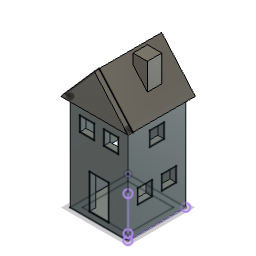
MMEZP_Domecek_2_patra v1 (Autodesk Fusion 360 design; units mm, degrees)
Autodesk Fusion 360 part; units mm, degrees
sketch "Sketch1" plane through (0, 0, 0) normal (0, 1, 0) x (1, 0, 0)
  line L0 (0, 0) -> (30, 0)
  line L1 (30, 0) -> (30, -30)
  line L2 (30, -30) -> (0, -30)
  line L3 (0, -30) -> (0, 0)
  line L4 (3.2, -3.2) -> (26.8, -3.2)
  line L5 (26.8, -3.2) -> (26.8, -26.8)
  line L6 (26.8, -26.8) -> (3.2, -26.8)
  line L7 (3.2, -26.8) -> (3.2, -3.2)
  dimension "d1" = 30
  dimension "d2" = 30
  dimension "d3" = 3.2
  dimension "d4" = 3.2
  dimension "d5" = 3.2
  dimension "d6" = 3.2
  constraint horizontal L0
  constraint vertical L1
  constraint horizontal L2
  constraint vertical L3
  constraint coincident L0.start L3.end
  constraint horizontal L4
  constraint vertical L5
  constraint horizontal L6
  constraint vertical L7
  measures "d1" distance of L0.start L0.end
  measures "d2" distance of L0.start L2.end
  measures "d3" distance of L1 L5
  measures "d4" distance of L0 L4
  measures "d5" distance of L3 L7
  measures "d6" distance of L2 L6
extrude "Extrude1" add sketch "Sketch1" along normal blind 50 makes body 1
sketch "Sketch2" plane through (0, 0, 30) normal (0, 0, 1) x (1, 0, 0)
  line L0 (0, 0) -> (30, 0)
  line L1 (30, 0) -> (30, 50)
  line L2 (30, 50) -> (0, 50)
  line L3 (0, 50) -> (0, 0)
  line L4 (10, 3.2) -> (20, 3.2)
  line L5 (20, 3.2) -> (20, 21.2)
  line L6 (20, 21.2) -> (10, 21.2)
  line L7 (10, 21.2) -> (10, 3.2)
  line L8 (5, 44) -> (12.5, 44)
  line L9 (12.5, 44) -> (12.5, 36.5)
  line L10 (12.5, 36.5) -> (5, 36.5)
  line L11 (5, 36.5) -> (5, 44)
  line L12 (17.5, 44) -> (25, 44)
  line L13 (25, 44) -> (25, 36.5)
  line L14 (25, 36.5) -> (17.5, 36.5)
  line L15 (17.5, 36.5) -> (17.5, 44)
  line L16 (0, 50) -> (-2.5, 50)
  line L17 (30, 50) -> (32.5, 50)
  line L18 (-2.5, 50) -> (15, 70)
  line L19 (15, 70) -> (32.5, 50)
  dimension "d9" = 18
  dimension "d10" = 10
  dimension "d11" = 10
  dimension "d12" = 3.2
  dimension "d13" = 7.5
  dimension "d14" = 7.5
  dimension "d15" = 5
  dimension "d16" = 6
  dimension "d17" = 7.5
  dimension "d18" = 7.5
  dimension "d19" = 5
  dimension "d20" = 6
  dimension "d51" = 2.5
  dimension "d52" = 2.5
  dimension "d53" = 17.5
  dimension "d54" = 20
  constraint horizontal L4
  constraint vertical L5
  constraint horizontal L6
  constraint vertical L7
  constraint horizontal L8
  constraint vertical L9
  constraint horizontal L10
  constraint vertical L11
  constraint horizontal L12
  constraint vertical L13
  constraint horizontal L14
  constraint vertical L15
  constraint coincident L2.end L3.start
  constraint perpendicular L3 L16
  constraint coincident L1.end L2.start
  constraint perpendicular L1 L17
  measures "d9" distance of L4.start L6.end
  measures "d10" distance of L4.start L4.end
  measures "d11" distance of L3 L7
  measures "d12" distance of L0 L4
  measures "d13" distance of L8.start L8.end
  measures "d14" distance of L8.start L10.end
  measures "d15" distance of L3 L11
  measures "d16" distance of L2 L8
  measures "d17" distance of L12.start L12.end
  measures "d18" distance of L12.start L14.end
  measures "d19" distance of L1 L13
  measures "d20" distance of L2 L12
  measures "d51" distance of L2.end L16.end
  measures "d52" distance of L1.end L17.end
  measures "d53" horizontal distance of L17.end L18.end
  measures "d54" distance of L2 L18.end
extrude "Extrude2" cut sketch "Sketch2" against normal blind 3.2 contours L4 L5 L6 L7 bodies 1
extrude "Extrude3" add sketch "Sketch1" along normal blind 3.2 contours L4 L5 L6 L7 bodies 1
extrude "Extrude4" cut sketch "Sketch2" against normal blind 3.2 contours L8 L9 L10 L11 | L12 L13 L14 L15 bodies 1
sketch "Sketch3" plane through (30, 0, 0) normal (1, 0, 0) x (0, 0, -1)
  line L0 (-30, 0) -> (0, 0)
  line L1 (0, 0) -> (0, 50)
  line L2 (0, 50) -> (-30, 50)
  line L3 (-30, 50) -> (-30, 0)
  line L4 (-25, 21.2) -> (-17.5, 21.2)
  line L5 (-17.5, 21.2) -> (-17.5, 13.7)
  line L6 (-17.5, 13.7) -> (-25, 13.7)
  line L7 (-25, 13.7) -> (-25, 21.2)
  line L8 (-12.5, 21.2) -> (-5, 21.2)
  line L9 (-5, 21.2) -> (-5, 13.7)
  line L10 (-5, 13.7) -> (-12.5, 13.7)
  line L11 (-12.5, 13.7) -> (-12.5, 21.2)
  line L12 (-30, 3.2) -> (-30, 21.2)
  line L13 (0, 0) -> (-30, 0)
  line L14 (-18.75, 44) -> (-11.25, 44)
  line L15 (-11.25, 44) -> (-11.25, 36.5)
  line L16 (-11.25, 36.5) -> (-18.75, 36.5)
  line L17 (-18.75, 36.5) -> (-18.75, 44)
  dimension "d27" = 7.5
  dimension "d28" = 7.5
  dimension "d29" = 5
  dimension "d30" = 5
  dimension "d31" = 7.5
  dimension "d32" = 7.5
  dimension "d33" = 13.7
  dimension "d34" = 13.7
  dimension "d35" = 6
  dimension "d36" = 7.5
  dimension "d37" = 7.5
  dimension "d38" = 11.25
  constraint horizontal L4
  constraint vertical L5
  constraint horizontal L6
  constraint vertical L7
  constraint horizontal L8
  constraint vertical L9
  constraint horizontal L10
  constraint vertical L11
  constraint horizontal L14
  constraint vertical L15
  constraint horizontal L16
  constraint vertical L17
  measures "d27" distance of L4.start L4.end
  measures "d28" distance of L4.start L6.end
  measures "d29" distance of L7 L12
  measures "d30" distance of L1 L9
  measures "d31" distance of L8.start L8.end
  measures "d32" distance of L8.start L10.end
  measures "d33" distance of L6 L13
  measures "d34" distance of L10 L13
  measures "d35" distance of L2 L14
  measures "d36" distance of L14.start L16.end
  measures "d37" distance of L15.end L16.end
  measures "d38" distance of L1 L15
extrude "Extrude5" cut sketch "Sketch3" against normal blind 30 contours L14 L15 L16 L17 bodies 1
extrude "Extrude6" cut sketch "Sketch3" against normal blind 30 contours L4 L5 L6 L7 | L8 L9 L10 L11 bodies 1
sketch "Sketch4" plane through (0, 50, 0) normal (0, 1, 0) x (-1, 0, 0)
  line L0 (-26.8, 26.8) -> (-3.2, 26.8)
  line L1 (-3.2, 26.8) -> (-3.2, 3.2)
  line L2 (-3.2, 3.2) -> (-26.8, 3.2)
  line L3 (-26.8, 3.2) -> (-26.8, 26.8)
  line L4 (0, 30) -> (-30, 30)
  line L5 (-30, 30) -> (-30, 0)
  line L6 (-30, 0) -> (0, 0)
  line L7 (0, 0) -> (0, 30)
  line L8 (2.5, -2.5) -> (-32.5, -2.5)
  line L9 (-32.5, -2.5) -> (-32.5, 32.5)
  line L10 (-32.5, 32.5) -> (2.5, 32.5)
  line L11 (2.5, 32.5) -> (2.5, -2.5)
  line L12 (0, 30) -> (0, 0)
  line L13 (0, 0) -> (-30, 0)
  line L14 (-30, 0) -> (-30, 30)
  line L15 (-30, 30) -> (0, 30)
  line L16 (-18.3, 8.2) -> (-25.8, 8.2)
  line L17 (-25.8, 8.2) -> (-25.8, 15.7)
  line L18 (-25.8, 15.7) -> (-18.3, 15.7)
  line L19 (-18.3, 15.7) -> (-18.3, 8.2)
  line L20 (-26.8, 26.8) -> (-3.2, 26.8)
  line L21 (-26.8, 3.2) -> (-26.8, 26.8)
  line L22 (-3.2, 3.2) -> (-26.8, 3.2)
  dimension "d43" = 2.5
  dimension "d44" = 2.5
  dimension "d45" = 2.5
  dimension "d46" = 2.5
  dimension "d47" = 7.5
  dimension "d48" = 7.5
  dimension "d59" = 1
  dimension "d60" = 5
  constraint horizontal L8
  constraint vertical L9
  constraint horizontal L10
  constraint vertical L11
  constraint horizontal L16
  constraint vertical L17
  constraint horizontal L18
  constraint vertical L19
  measures "d43" distance of L11 L12
  measures "d44" distance of L8 L13
  measures "d45" distance of L9 L14
  measures "d46" distance of L10 L15
  measures "d47" distance of L16.start L16.end
  measures "d48" distance of L16.end L17.end
  measures "d59" distance of L17 L21
  measures "d60" distance of L16 L22
extrude "Extrude7" add sketch "Sketch2" along normal blind 2.5 separate body contours L2 L16 L17 L18 L19 makes body 2
extrude "Extrude8" add sketch "Sketch2" against normal blind 32.5 contours L2 L16 L17 L18 L19 bodies 1 2
extrude "Extrude9" add sketch "Sketch4" along normal blind 21.5 contours L16 L17 L18 L19 bodies 1
